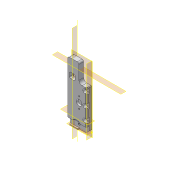
# Autodesk Inventor part: J002875
Saved by Autodesk Inventor 2012 SP2 (Build 160219200, 219)
## iProperties
Created: 2014-07-28
Material: ALUMINUM, 6061-T651
Vendor: HHMI: JFRC - ID&F
Document SubType Name: Modeling
Designer: arnoldj
Density: 2.7 g/cm^3
Part Number: J002875
Description: MPS Top Plate Right
Mass: 84.1919 g
Surface Area: 117.677 cm^2
Volume: 31.1822 cm^3
Project: P-194005
RuleStatus: InUse
AfterDocSave0: file://Part Number Cleaner
LAB/DEPT: SVOBODA (LAB)
REQUESTING SCIENTIST: PERON, SIMON
SURFACE ROUGHNESS: 63 Ra
DESIGN DEPARTMENT: HHMI: JFRC - ID&F
SPECIAL FINISH: ANODIZE PER MIL-A-8625F, TYPE II, CLASS 2 (BLACK)
ALTERED ITEM PART NUMBER: N/A
ALTERED ITEM VENDOR: N/A
ALTERED ITEM DESCRIPTION: N/A
Revision Number: -
Autodesk Inventor part; units mm, degrees
ref_plane "Work Plane1-between two actuators" through (-29.0322, 0, 0) normal (1, 0, 0) x (0, 1, 0)
ref_plane "Work Plane2-Y position of rear act" through (0, 105.283, 0) normal (0, 1, 0) x (-1, 0, 0)
ref_plane "Work Plane5-Y Position of Front Actuator" through (0, 18.923, 0) normal (0, 1, 0) x (-1, 0, 0)
ref_plane "Work Plane3-top of part" through (0, 0, 9.525) normal (0, 0, 1) x (1, 0, 0)
ref_plane "Work Plane4 -Assembly Mate Height" through (0, 0, -0.8636) normal (0, 0, 1) x (1, 0, 0)
ref_plane "Work Plane6 center of ball tip plane" through (0, 0, -0.2794) normal (0, 0, 1) x (1, 0, 0)
sketch "Sketch5" plane through (0, 0, 0) normal (1, 0, 0) x (0, 1, 0)
  point P0 (0, 0)
sketch "Sketch1" plane through (0, 0, 0) normal (0, 0, 1) x (1, 0, 0)
  line L0 (-38.1, 117.7798) -> (0, 117.7798)
  line L1 (0, 117.7798) -> (0, -2.5908)
  line L2 (-38.1, -2.5908) -> (-38.1, 117.7798)
  line L3 (-38.1, -2.5908) -> (0, -2.5908)
  line L4 (-45.72, 0) -> (7.62, 0) projected
  line L5 (0, 142.0481) -> (0, -27.8299) projected
  point P0 (0, 0)
  point P1 (0, -3.5617)
  dimension "d0" = 38.1
  dimension "d55" = 0
  dimension "d135" = 117.7798
  dimension "d136" = 2.5908
  constraints: 8 end point, 2 perpendicular, 1 horizontal, 1 parallel, 1 vertical alignment
  measures "d0" distance of L1.end L2.start
  measures "d55" distance between parallel lines of L1 L5
  measures "d135" distance between parallel lines of L4 L0
  measures "d136" distance between parallel lines of L4 L3
extrude "Extrusion1" add sketch "Sketch1" along normal blind 9.525
sketch "Sketch9" plane through (0, 0, 0) normal (0, 0, 1) x (1, 0, 0)
  circle A0 centre (-3.81, 65.7098) radius 1.6002
  circle A1 centre (-3.81, 14.9098) radius 1.6002
  line L0 (0, 117.7798) -> (0, 0) projected
  line L1 (-6.4922, 0) -> (1.082, 0) projected
  circle A2 centre (-3.81, 67.31) radius 1.6002
  circle A3 centre (-3.81, 64.1096) radius 1.6002
  line L2 (-5.4102, 67.31) -> (-5.4102, 64.1096)
  line L3 (-2.2098, 67.31) -> (-2.2098, 64.1096)
  line L4 (-3.81, 65.7098) -> (-3.81, 14.9098)
  dimension "d59" = 3.2004
  dimension "d60" = 3.2004
  dimension "d61" = 50.8
  dimension "d62" = 3.81
  dimension "d63" = 14.9098
  constraints: 6 end point, 6 point on circle, 4 centre point, 2 equal radius, 2 tangent, 1 parallel, 1 vertical alignment
  measures "d59" diameter of A0
  measures "d60" diameter of A1
  measures "d61" distance of L4.end L4.start
  measures "d62" distance from line of L4.start L0
  measures "d63" distance from line of L4.end L1
extrude "Locating Pin features Extrusion7" cut sketch "Sketch9" along normal blind 6.35
sketch "Sketch10" plane through (0, 0, 9.525) normal (0, 0, 1) x (1, 0, 0)
  circle A0 centre (-3.81, 14.9098) radius 1.6002 projected
  circle A1 centre (-3.81, 23.1648) radius 1.5875
  circle A2 centre (-3.81, 73.9648) radius 1.5875
  arc A3 (-2.2098, 67.31) -> (-5.4102, 67.31) centre (-3.81, 67.31) ccw projected
  arc A4 (-5.4102, 64.1096) -> (-2.2098, 64.1096) centre (-3.81, 64.1096) ccw projected
  line L0 (-5.4102, 64.1096) -> (-5.4102, 67.31) projected
  line L1 (-2.2098, 67.31) -> (-2.2098, 64.1096) projected
  line L2 (-5.4102, 65.7098) -> (-2.2098, 65.7098)
  line L3 (-3.81, 65.7098) -> (-3.81, 14.9098)
  point P0 (0, 0)
  point P1 (-3.81, 48.5648)
  dimension "d67" = 3.175
  dimension "d68" = 3.175
  dimension "d69" = 50.8
  dimension "d282" = 23.1648
  dimension "d295" = 25.4
  constraints: 4 end point, 3 midpoint, 2 centre point, 2 vertical alignment, 1 perpendicular, 1 point on line
  measures "d67" diameter of A2
  measures "d68" diameter of A1
  measures "d69" distance of A2.centre A1.centre
  measures "d282" vertical distance of point (0, 0) A1.centre
  measures "d295" distance of point (-3.81, 48.565) A2.centre
hole "Mtg Holes Hole2" at (-3.81, 23.1648, 9.525) at (-3.81, 73.9648, 9.525) at (-3.81, 48.5648, 9.525) direction (0, 0, -1) diameter 4.4958 end through all
sketch "Sketch22" plane through (0, 0, 0) normal (0, 0, 1) x (1, 0, 0)
  circle A0 centre (-29.0418, 18.923) radius 2.54 construction
  line L0 (-41.6966, 105.283) -> (6.9494, 105.283) construction
  line L1 (-34.7472, 93.218) -> (-23.3172, 93.218)
  line L2 (-23.3172, 93.218) -> (-23.3172, 81.788)
  line L3 (-23.3172, 81.788) -> (-34.7472, 81.788)
  line L4 (-34.7472, 81.788) -> (-34.7472, 93.218)
  line L5 (-23.3172, 87.503) -> (-34.7472, 87.503) construction
  line L6 (-34.7472, 38.608) -> (-23.3172, 38.608)
  line L7 (-23.3172, 38.608) -> (-23.3172, 27.178)
  line L8 (-23.3172, 27.178) -> (-34.7472, 27.178)
  line L9 (-34.7472, 27.178) -> (-34.7472, 38.608)
  line L10 (-23.3172, 32.893) -> (-34.7472, 32.893) construction
  line L11 (-41.6966, 18.923) -> (6.9494, 18.923) projected
  line L12 (-29.0322, 111.8616) -> (-29.0322, -18.6436) projected
  line L13 (-29.0322, 93.218) -> (-29.0322, 81.788) construction
  line L14 (-29.0322, 93.218) -> (-29.0322, 81.788) construction
  line L15 (-29.0322, 38.608) -> (-29.0322, 27.178) construction
  dimension "d149" = 11.43
  dimension "d150" = 11.43
  dimension "d225" = 13.97
  dimension "d226" = 17.78
  dimension "d227" = 0
  constraints: 26 end point, 10 midpoint, 4 parallel, 2 equal length, 2 horizontal, 2 perpendicular, 2 point on line, 1 vertical alignment
  measures "d149" distance of L2.end L3.end
  measures "d150" distance of L1.end L2.end
  measures "d225" distance between parallel lines of L10 L11
  measures "d226" distance between parallel lines of L5 L0
  measures "d227" distance between parallel lines of L12 L14
extrude "Extrusion13" cut sketch "Sketch22" along normal through all contours L1 L12 L3 L4 | L1 L2 L3 L12
sketch "Sketch38" plane through (0, 0, 9.525) normal (0, 0, 1) x (1, 0, 0)
  line L0 (-38.1, -2.5908) -> (-38.1, 117.7798) projected
  line L1 (0, -2.5908) -> (-38.1, -2.5908) projected
  line L2 (-38.1, -0.6858) -> (0, -0.6858)
  line L3 (0, -0.6858) -> (0, 12.065)
  line L4 (0, 12.065) -> (-38.1, 12.065)
  line L5 (-38.1, 12.065) -> (-38.1, -0.6858)
  line L6 (-20.1422, -0.6858) -> (0, -0.6858)
  line L7 (0, -0.6858) -> (0, -2.5908)
  line L8 (0, -2.5908) -> (-20.1422, -2.5908)
  line L9 (-20.1422, -2.5908) -> (-20.1422, -0.6858)
  point P0 (0, 0)
  dimension "d302" = 17.9578
  dimension "d303" = 1.905
  dimension "d304" = 12.7508
  constraints: 16 end point, 4 parallel, 2 horizontal, 2 perpendicular, 2 point on line, 1 vertical alignment
  measures "d302" distance between parallel lines of L9 L0
  measures "d303" distance between parallel lines of L1 L2
  measures "d304" distance between parallel lines of L2 L4
extrude "Extrusion22" cut sketch "Sketch38" against normal blind 5.6134 contours L0 L4 L3 L2 | L9 L2 L7 L1
sketch "Sketch39" plane through (0, 0, 0) normal (0, 0, 1) x (1, 0, 0)
  line L0 (-38.1, -0.6858) -> (-38.1, 12.065) projected
  line L1 (-38.1, 12.065) -> (0, 12.065) projected
  point P0 (0, 0)
  point P1 (-20.955, 5.6896)
  dimension "d307" = 17.145
  dimension "d308" = 6.3754
  measures "d307" distance from line of point (-20.955, 5.69) L0
  measures "d308" distance from line of point (-20.955, 5.69) L1
hole "Hole10" at (-20.955, 5.6896, 0) direction (0, 0, 1) diameter 4.1402 end through all
sketch "Sketch40" plane through (0, 0, 9.525) normal (0, 0, 1) x (1, 0, 0)
  line L0 (-20.1422, -0.6858) -> (-38.1, -0.6858) projected
  line L1 (-38.1, -2.5908) -> (-38.1, -0.6858) projected
  line L2 (-20.1422, -2.5908) -> (-20.1422, -0.6858) projected
  line L3 (-20.1422, -2.5908) -> (-38.1, -2.5908) projected
  circle A0 centre (-20.955, 5.6896) radius 2.0701 projected
  line L4 (-38.1, -0.6858) -> (-20.1422, -0.6858)
  line L5 (-20.1422, -0.6858) -> (-20.1422, -2.5908)
  line L6 (-20.1422, -2.5908) -> (-38.1, -2.5908)
  line L7 (-38.1, -2.5908) -> (-38.1, -0.6858)
  circle A1 centre (-20.955, 5.6896) radius 9.525
  point P0 (0, 0)
  dimension "d316" = 19.05
  constraints: 8 end point, 2 parallel, 1 centre point, 1 coincident, 1 horizontal, 1 perpendicular
  measures "d316" diameter of A1
extrude "Extrusion23" cut sketch "Sketch40" against normal blind 2.4384 contours L2 L3 A1 L0 | L0 A1 L3 L2 | A1 L3 L1 L0 | A0
sketch "Sketch34" plane through (0, 0, 9.525) normal (0, 0, 1) x (1, 0, 0)
  circle A0 centre (-3.81, 73.9648) radius 2.2479 projected
  circle A1 centre (-3.81, 23.1648) radius 2.2479 projected
  line L0 (0, 117.7798) -> (0, -2.5908) projected
  line L1 (0, -2.5908) -> (-38.1, -2.5908) projected
  line L2 (-3.81, 73.9648) -> (-3.81, 23.1648)
  line L3 (-15.4375, 59.5648) -> (-15.4375, 37.5648)
  line L4 (0, 141.8539) -> (0, -26.6649) projected
  point P0 (0, 0)
  point P1 (-15.4375, 48.5648)
  point P2 (-3.81, 48.5648)
  dimension "d269" = 22
  dimension "d270" = 15.4375
  constraints: 4 end point, 2 coincident, 2 midpoint, 1 horizontal alignment, 1 parallel, 1 perpendicular
  measures "d269" distance of L3.start L3.end
  measures "d270" distance between parallel lines of L0 L3
hole "Hole9" at (-15.4375, 59.5648, 9.525) at (-15.4375, 37.5648, 9.525) direction (0, 0, -1) diameter 2.4638 end through all
fillet "Fillet10" radius 2.54 4 edges at (-23.3172, 93.218, 4.7625) (-23.3172, 81.788, 4.7625) (-34.7472, 81.788, 4.7625) (-34.7472, 93.218, 4.7625)
sketch "Sketch24" plane through (0, 0, 0) normal (0, 0, 1) x (1, 0, 0)
  circle A0 centre (-32.8422, 76.708) radius 1.27
  circle A1 centre (-25.2222, 76.708) radius 1.27
  line L0 (-41.6966, 105.283) -> (6.9494, 105.283) projected
  line L1 (-34.7472, 84.328) -> (-34.7472, 90.678) construction
  line L2 (-34.7472, 87.503) -> (-31.3197, 87.503) construction
  line L3 (-29.0322, 170.9362) -> (-29.0322, -28.4894) construction
  line L4 (-29.0322, 105.283) -> (-29.0322, 142.4468) construction
  dimension "d167" = 2.54
  dimension "d168" = 7.62
  dimension "d236" = 10.795
  constraints: 4 end point, 3 point on line, 2 centre point, 1 equal radius, 1 horizontal alignment, 1 midpoint, 1 perpendicular, 1 symmetric about line
  measures "d167" diameter of A0
  measures "d168" distance of A1.centre A0.centre
  measures "d236" distance from line of L2 A0.centre
hole "Hole4" [suppressed]
sketch "Sketch31" plane through (0, 0, 9.525) normal (0, 0, 1) x (1, 0, 0)
  line L0 (-45.72, 105.283) -> (7.62, 105.283) projected
  line L1 (-29.0322, 141.8539) -> (-29.0322, -26.6649) projected
  point P0 (0, 0)
  point P1 (-29.0322, 105.283)
  constraints: 2 point on line
hole "Hole6" [suppressed]
sketch "Sketch33" plane through (0, 0, 0) normal (0, 0, -1) x (-1, 0, 0)
  line L0 (-7.62, 105.283) -> (45.72, 105.283) projected
  line L1 (29.0322, -26.6649) -> (29.0322, 141.8539) projected
  point P0 (0, 0)
  point P1 (29.0322, 105.283)
  constraints: 2 point on line
hole "Hole8" at (-29.0322, 105.283, 0) direction (0, 0, 1) diameter 13.081 depth 4.5466 counterbore diameter 15.875 counterbore depth 2.54
sketch "Sketch44" plane through (0, 0, 0) normal (0, 0, -1) x (-1, 0, 0)
  circle A0 centre (25.2222, 76.708) radius 1.2319 projected
  circle A1 centre (32.8422, 76.708) radius 1.2319 projected
  line L0 (23.3172, 84.328) -> (23.3172, 90.678) projected
  arc A2 (25.8572, 93.218) -> (23.3172, 90.678) centre (25.8572, 90.678) ccw projected
  line L1 (25.8572, 93.218) -> (32.2072, 93.218) projected
  line L2 (34.7472, 90.678) -> (34.7472, 84.328) projected
  line L3 (32.2072, 81.788) -> (25.8572, 81.788) projected
  line L4 (23.3172, 90.678) -> (34.7472, 90.678)
  line L5 (34.7472, 90.678) -> (34.7472, 72.898)
  line L6 (34.7472, 72.898) -> (23.3172, 72.898)
  line L7 (23.3172, 72.898) -> (23.3172, 90.678)
  point P0 (0, 0)
  dimension "d341" = 8.89
  constraints: 8 end point, 2 coincident, 2 parallel, 1 horizontal, 1 horizontal alignment, 1 perpendicular
  measures "d341" distance between parallel lines of L6 L3
extrude "Extrusion24" cut sketch "Sketch44" against normal blind 2.54 contours A0 | A1 | L0 L4 L2 L5 L6 L7
fillet "Fillet27" radius 2.54 2 edges at (-23.3172, 72.898, 1.27) (-34.7472, 72.898, 1.27)
chamfer "Chamfer17" distance 0.635 angle 45 8 edges at (-23.3172, 83.058, 0) (-24.0611, 92.4741, 0) (-29.0322, 93.218, 0) (-34.0033, 92.4741, 0) (-34.7472, 83.058, 0) (-34.0033, 73.6419, 0) (-29.0322, 72.898, 0) (-24.0611, 73.6419, 0)
sketch "Sketch35" plane through (0, 0, 0) normal (0, 0, 1) x (1, 0, 0)
  line L0 (-38.1, 117.7798) -> (0, 117.7798) projected
  line L1 (0, 117.7798) -> (0, 12.065) projected
  line L2 (0, 117.7798) -> (-15.875, 117.7798)
  line L3 (-15.875, 117.7798) -> (-15.875, 80.9498)
  line L4 (-15.875, 80.9498) -> (0, 80.9498)
  line L5 (0, 80.9498) -> (0, 117.7798)
  line L6 (-38.1, 12.065) -> (-38.1, 117.7798) projected
  point P0 (0, 0)
  point P1 (0, 4.3942)
  point P2 (-38.1, -2.5908)
  point P3 (0, 1.8542)
  point P4 (0, -2.5908)
  dimension "d283" = 15.875
  dimension "d284" = 22.225
  dimension "d285" = 36.83
  constraints: 8 end point, 2 parallel, 1 horizontal, 1 perpendicular
  measures "d283" distance of L0.end L2.end
  measures "d284" distance between parallel lines of L3 L6
  measures "d285" distance of L2.end L3.end
extrude "Extrusion19" cut sketch "Sketch35" along normal blind 25.4
sketch "Sketch37" plane through (0, 0, 9.525) normal (0, 0, 1) x (1, 0, 0)
  circle A0 centre (-3.81, 48.5648) radius 2.2479 projected
  circle A1 centre (-3.81, 73.9648) radius 2.2479 projected
  circle A2 centre (-3.81, 23.1648) radius 2.2479 projected
  circle A3 centre (-3.81, 73.9648) radius 4.1275
  circle A4 centre (-3.81, 48.5648) radius 4.1275
  circle A5 centre (-3.81, 23.1648) radius 4.1275
  line L0 (-3.81, 78.0923) -> (0.3175, 78.0923)
  line L1 (0.3175, 78.0923) -> (0.3175, 69.8373)
  line L2 (0.3175, 69.8373) -> (-3.81, 69.8373)
  line L3 (-3.81, 69.8373) -> (-3.81, 78.0923)
  line L4 (-3.81, 52.6923) -> (0.3175, 52.6923)
  line L5 (0.3175, 52.6923) -> (0.3175, 44.4373)
  line L6 (0.3175, 44.4373) -> (-3.81, 44.4373)
  line L7 (-3.81, 44.4373) -> (-3.81, 52.6923)
  line L8 (-3.81, 27.2923) -> (0.3175, 27.2923)
  line L9 (0.3175, 27.2923) -> (0.3175, 19.0373)
  line L10 (0.3175, 19.0373) -> (-3.81, 19.0373)
  line L11 (-3.81, 19.0373) -> (-3.81, 27.2923)
  point P0 (0, 0)
  dimension "d298" = 8.255
  constraints: 24 end point, 6 horizontal, 6 parallel, 3 coincident, 3 perpendicular, 3 vertical, 3 vertical alignment, 6 other
extrude "Extrusion21" cut sketch "Sketch37" against normal blind 5.715 contours A0 L7 | A0 L7 A4 | A0 L7 A4 | L4 L5 A4 | A4 L5 L6 | A1 L3 | A1 L3 A3 | A1 L3 A3 | L0 L1 A3 | A3 L1 L2 | A2 L11 | A2 L11 A5 | A2 L11 A5 | L8 L9 A5 | A5 L9 L10 picked at (-2.5903, 49.1767) picked at (-3.3428, 74.5506) picked at (-3.0093, 23.7506)
chamfer "Chamfer12" distance 0.635 angle 45 1 edges at (-29.0322, 97.3455, 0)
fillet "Fillet20" radius 6.35 1 edges at (-15.875, 80.9498, 4.7625)
fillet "Fillet21" radius 3.175 2 edges at (-15.875, 117.7798, 4.7625) (-38.1, 117.7798, 4.7625)
fillet "Fillet23" [suppressed]
chamfer "Chamfer13" distance 1.905 angle 45 2 edges at (-20.1422, -1.6383, 7.0866) (-38.1, -1.6383, 7.0866)
chamfer "Chamfer14" distance 6.985 angle 45 1 edges at (0, -2.5908, 1.9558)
fillet "Fillet24" radius 1.27 2 edges at (0, 4.3942, 1.9558) (-6.985, -2.5908, 1.9558)
chamfer "Chamfer15" distance 0.635 angle 45 1 edges at (-20.955, 15.2146, 9.525)
fillet "Fillet25" radius 1.27 2 edges at (-13.8783, 12.065, 7.9883) (-28.0317, 12.065, 7.9883)
chamfer "Chamfer16" distance 3.175 angle 45 4 edges at (0, 15.5512, 9.525) (0, 35.8648, 9.525) (0, 61.2648, 9.525) (0, 79.5211, 9.525)
fillet "Fillet26" radius 1.27 8 edges at (0, 12.065, 5.1308) (0, 19.0373, 5.08) (0, 27.2923, 5.08) (0, 44.4373, 5.08) (0, 52.6923, 5.08) (0, 69.8373, 5.08) (0, 78.0923, 5.08) (0, 80.9498, 3.175)
sketch "Sketch41" plane through (0, 0, 9.525) normal (0, 0, 1) x (1, 0, 0)
  circle A0 centre (-15.4375, 37.5648) radius 1.2319 projected
  circle A1 centre (-15.4375, 59.5648) radius 1.2319 projected
  line L0 (-32.2072, 93.218) -> (-25.8572, 93.218) projected
  line L1 (-15.4375, 59.5648) -> (-15.4375, 37.5648) construction
  point P0 (0, 0)
  point P1 (-15.4375, 48.5648)
  constraints: 2 end point, 1 midpoint, 1 perpendicular
hole "Hole11" at (-15.4375, 48.5648, 9.525) direction (0, 0, -1) diameter 11.43 depth 3.81
fillet "Fillet28" radius 1.27 1 edges at (-38.1, 12.065, 6.7183)
body "Solid1"
